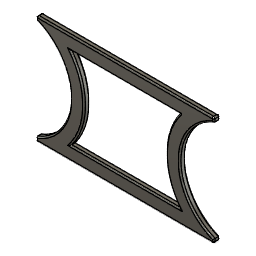
Flight Stand Huge (Autodesk Fusion 360 design; units mm, degrees)
Autodesk Fusion 360 part; units mm, degrees
note: some values were not read from the file. Chosen so that the rebuilt part matches the saved one: which face or edge a step refers to. Set by a fixed rule: which sketch regions a step uses.
sketch "Sketch1" plane through (0, 0, 0) normal (0, 0, 1) x (1, 0, 0)
  line L0 (0, 0) -> (65, 0)
  line L1 (0, 40) -> (65, 40)
  line L2 (32.5, 40) -> (32.5, 0) construction
  line L3 (12.5, 20) -> (52.5, 20) construction
  line L4 (0, 40) -> (0, 38.5)
  line L5 (65, 40) -> (65, 38.5)
  line L6 (65, 0) -> (65, 1.5)
  line L7 (0, 0) -> (0, 1.5)
  arc A0 (0, 1.5) -> (0, 38.5) centre (-7.44, 20) ccw
  arc A1 (65, 38.5) -> (65, 1.5) centre (72.44, 20) ccw
  dimension "d1" = 65
  dimension "d4" = 40
  dimension "d8" = 1.5
  dimension "d9" = 40
  constraint coincident L0.start L7.start
  constraint horizontal L1
  constraint midpoint L1 L2.start
  constraint midpoint L0 L2.end
  constraint midpoint L2 L3
  constraint perpendicular L1 L4
  constraint perpendicular L1 L5
  constraint equal L0 L1
  constraint horizontal L0
  constraint equal L6 L7
  constraint equal L5 L6
  constraint equal L4 L5
  constraint collinear L4 L7
  constraint coincident L3.start A0
  constraint horizontal L3
  constraint perpendicular L0 L6
  constraint coincident L3.end A1
  measures "d1" distance of L0.start L0.end
  measures "d4" distance of L3.start L3.end
  measures "d8" distance of L0.start L7.end
  measures "d9" distance of L0 L1
extrude "Extrude1" add sketch "Sketch1" along normal blind 2.2
sketch "Sketch3" plane through (0, 0, 2.2) normal (0, 0, 1) x (1, 0, 0)
  line L0 (0, 40) -> (0, 38.5)
  arc A0 (0, 1.5) -> (0, 38.5) centre (-7.44, 20) ccw
  line L1 (0, 1.5) -> (0, 0)
  line L2 (0, 0) -> (65, 0)
  line L3 (65, 0) -> (65, 1.5)
  arc A1 (65, 38.5) -> (65, 1.5) centre (72.44, 20) ccw
  line L4 (65, 38.5) -> (65, 40)
  line L5 (65, 40) -> (0, 40)
  line L6 (12.5, 35) -> (52.5, 35)
  line L7 (52.5, 5) -> (12.5, 5)
  line L8 (0, 40) -> (65, 40)
  line L9 (0, 0) -> (65, 0)
  line L10 (32.5, 0) -> (32.5, 40)
  line L11 (27, 20) -> (17.512, 20)
  line L12 (17.512, 20) -> (47.488, 20)
  arc A2 (52.5, 35) -> (52.5, 5) centre (72.44, 20) ccw
  arc A3 (12.5, 5) -> (12.5, 35) centre (-7.44, 20) ccw
  point P0 (32.5, 35)
  point P1 (32.5, 5)
  point P2 (32.5, 20)
  dimension "d10" = 5
  dimension "d11" = 5
  dimension "d13" = 40
  constraint horizontal L6
  constraint horizontal L7
  constraint equal L6 L7
  constraint midpoint L9 L10.start
  constraint midpoint L8 L10.end
  constraint coincident L10 P0
  constraint coincident L6 P0
  constraint midpoint L7 P1
  constraint midpoint L6 P0
  constraint horizontal L11
  constraint perpendicular L10 L12
  constraint midpoint L10 P2
  constraint coincident L12 P2
  constraint midpoint L12 P2
  constraint coincident L12.end A2
  constraint coincident L11.end A3
  constraint coincident L10 P1
  constraint coincident A0.centre A3.centre
  measures "d10" distance of L6 L8
  measures "d11" distance of L7 L9
  measures "d13" distance of L7.start L7.end
extrude "Extrude2" cut sketch "Sketch3" against normal blind 5 contours L6 L10 L11 L12 A3 | L6 L10 L12 A2 | L7 L10 L12 A2 | L7 L10 L11 L12 A3
fillet "Fillet1" radius 0.5 28 edges at (0, 0, 1.1) (0, 0.75, 0) (0, 0.75, 2.2) (65, 0, 1.1) (32.5, 0, 0) (32.5, 0, 2.2) (12.5, 20, 0) (12.5, 20, 2.2) (65, 0.75, 0) (52.5, 20, 0) (65, 39.25, 0) (32.5, 40, 0) (0, 39.25, 0) (17.512, 20, 0) (32.5, 35, 0) (47.488, 20, 0) (32.5, 5, 0) (65, 0.75, 2.2) (52.5, 20, 2.2) (65, 39.25, 2.2) (32.5, 40, 2.2) (0, 39.25, 2.2) (32.5, 35, 2.2) (47.488, 20, 2.2) (32.5, 5, 2.2) (17.512, 20, 2.2) (0, 40, 1.1) (65, 40, 1.1)
named bodies: "Flight Stand Huge"
